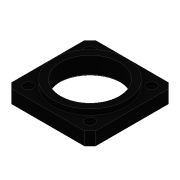
# Autodesk Inventor part: Festlager Deckel
Saved by Autodesk Inventor 2016 (Build 200138000, 138)
## iProperties
Created: 2015-07-27
Part Number: Festlager Deckel
Material: Aluminum 6061
Document SubType Name: Modeling
Density: 2.7 g/cm^3
Appearance: Smooth - Black
Autodesk Inventor part; units mm, degrees
ref_plane "YZ Plane" through (0, 0, 0) normal (1, 0, 0) x (0, 1, 0)
ref_plane "XZ Plane" through (0, 0, 0) normal (0, 1, 0) x (-1, 0, 0)
ref_plane "XY Plane" through (0, 0, 0) normal (0, 0, 1) x (1, 0, 0)
sketch "Sketch1" plane through (0, 0, 0) normal (0, 0, 1) x (1, 0, 0)
  line L0 (-15, -15) -> (15, -15)
  line L1 (15, -15) -> (15, 15)
  line L2 (15, 15) -> (-15, 15)
  line L3 (-15, 15) -> (-15, -15)
  line L4 (-15, -15) -> (15, 15) construction
  line L5 (15, -15) -> (-15, 15) construction
  point P0 (0, 0)
  dimension "d0" = 30
  dimension "d1" = 30
  constraints: 12 end point, 2 midpoint, 2 parallel, 1 horizontal, 1 perpendicular
  measures "d0" distance of L2.end L1.end
  measures "d1" distance of L1.end L0.end
extrude "Extrusion1" add sketch "Sketch1" along normal blind 4.7
sketch "Sketch2" plane through (0, 0, 4.7) normal (0, 0, 1) x (1, 0, 0)
  point P0 (0, 0)
hole "Hole1" at (0, 0, 4.7) direction (0, 0, -1) diameter 21 end through all
sketch "Sketch3" plane through (0, 0, 0) normal (0, 1, 0) x (-1, 0, 0)
  line L0 (-10.5, 6.7) -> (-13, 6.7)
  line L1 (-13, 6.7) -> (-13, 4.7)
  line L2 (-13, 4.7) -> (-10.5, 4.7)
  line L3 (-10.5, 4.7) -> (-10.5, 6.7)
  line L4 (-15, 4.7) -> (15, 4.7) projected
  line L5 (-10.5, 0) -> (-10.5, 4.7) projected
  line L6 (0, 0) -> (0, 4.7)
  line L7 (10.5, 0) -> (-10.5, 0) projected
  dimension "d13" = 26
  dimension "d15" = 2
  constraints: 10 end point, 2 collinear, 2 parallel, 1 horizontal, 1 midpoint, 1 perpendicular
  measures "d13" diameter of L1 L6
  measures "d15" distance between parallel lines of L4 L0
revolve "Revolution1" add sketch "Sketch3" angle 360 about axis through (0, 0, 0) along (0, 0, 1) contours L3 L2 L1 L0
sketch "Sketch4" plane through (0, 0, 0) normal (0, 0, -1) x (-1, 0, 0)
  line L0 (-11, -11) -> (11, -11)
  line L1 (11, -11) -> (11, 11)
  line L2 (11, 11) -> (-11, 11)
  line L3 (-11, 11) -> (-11, -11)
  line L4 (-11, -11) -> (11, 11) construction
  line L5 (11, -11) -> (-11, 11) construction
  point P0 (0, 0)
  point P1 (0, 0)
  dimension "d17" = 22
  constraints: 12 end point, 2 parallel, 2 perpendicular, 1 coincident, 1 horizontal, 1 midpoint
  measures "d17" distance of L1.end L2.end
hole "Hole2" at (11, 11, 0) at (-11, 11, 0) at (-11, -11, 0) at (11, -11, 0) direction (0, 0, 1) diameter 3.4 end through all counterbore diameter 6.5 counterbore depth 3.4
chamfer "Chamfer1" distance 2 angle 45 4 edges at (15, -15, 2.35) (15, 15, 2.35) (-15, 15, 2.35) (-15, -15, 2.35)
chamfer "Chamfer2" distance 0.7 angle 45 1 edges at (0, 10.5, 0)
body "Solid1"
